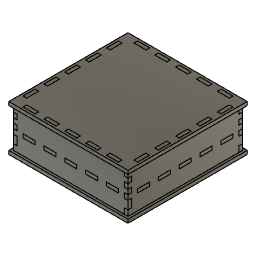
InfinityMirror (Autodesk Fusion 360 design; units mm, degrees)
Autodesk Fusion 360 part; units mm, degrees
sketch "Skizze1" plane through (0, 0, 0) normal (0, 0, 1) x (1, 0, 0) in component "Deckel"
  line L0 (50, -50) -> (-50, -50)
  line L1 (-50, -50) -> (-50, 50)
  line L2 (-50, 50) -> (50, 50)
  line L3 (50, 50) -> (50, -50)
  line L4 (50, -50) -> (-50, 50) construction
  line L5 (-50, -50) -> (50, 50) construction
  line L6 (45, -45) -> (-45, -45) construction
  line L7 (-45, -45) -> (-45, 45) construction
  line L8 (-45, 45) -> (45, 45) construction
  line L9 (45, 45) -> (45, -45) construction
  line L10 (45, -45) -> (-45, 45) construction
  line L11 (-45, -45) -> (45, 45) construction
  line L12 (-40, 45) -> (-30, 45)
  line L13 (-30, 45) -> (-30, 48)
  line L14 (-30, 48) -> (-40, 48)
  line L15 (-40, 48) -> (-40, 45)
  line L16 (-22.5, 45) -> (-12.5, 45)
  line L17 (-12.5, 45) -> (-12.5, 48)
  line L18 (-22.5, 48) -> (-22.5, 45)
  line L19 (-12.5, 48) -> (-22.5, 48)
  line L20 (-5, 45) -> (5, 45)
  line L21 (5, 45) -> (5, 48)
  line L22 (-5, 48) -> (-5, 45)
  line L23 (5, 48) -> (-5, 48)
  line L24 (12.5, 45) -> (22.5, 45)
  line L25 (22.5, 45) -> (22.5, 48)
  line L26 (12.5, 48) -> (12.5, 45)
  line L27 (22.5, 48) -> (12.5, 48)
  line L28 (30, 45) -> (40, 45)
  line L29 (40, 45) -> (40, 48)
  line L30 (30, 48) -> (30, 45)
  line L31 (40, 48) -> (30, 48)
  line L32 (-45, -22.5) -> (-45, -12.5)
  line L33 (-45, -12.5) -> (-48, -12.5)
  line L34 (-48, -12.5) -> (-48, -22.5)
  line L35 (-48, -22.5) -> (-45, -22.5)
  line L36 (-45, -40) -> (-45, -30)
  line L37 (-45, -30) -> (-48, -30)
  line L38 (-48, -40) -> (-45, -40)
  line L39 (-48, -30) -> (-48, -40)
  line L40 (-45, -5) -> (-45, 5)
  line L41 (-45, 5) -> (-48, 5)
  line L42 (-48, -5) -> (-45, -5)
  line L43 (-48, 5) -> (-48, -5)
  line L44 (-45, 12.5) -> (-45, 22.5)
  line L45 (-45, 22.5) -> (-48, 22.5)
  line L46 (-48, 12.5) -> (-45, 12.5)
  line L47 (-48, 22.5) -> (-48, 12.5)
  line L48 (-45, 30) -> (-45, 40)
  line L49 (-45, 40) -> (-48, 40)
  line L50 (-48, 30) -> (-45, 30)
  line L51 (-48, 40) -> (-48, 30)
  line L52 (22.5, -45) -> (12.5, -45)
  line L53 (12.5, -45) -> (12.5, -48)
  line L54 (12.5, -48) -> (22.5, -48)
  line L55 (22.5, -48) -> (22.5, -45)
  line L56 (40, -45) -> (30, -45)
  line L57 (30, -45) -> (30, -48)
  line L58 (40, -48) -> (40, -45)
  line L59 (30, -48) -> (40, -48)
  line L60 (5, -45) -> (-5, -45)
  line L61 (-5, -45) -> (-5, -48)
  line L62 (5, -48) -> (5, -45)
  line L63 (-5, -48) -> (5, -48)
  line L64 (-12.5, -45) -> (-22.5, -45)
  line L65 (-22.5, -45) -> (-22.5, -48)
  line L66 (-12.5, -48) -> (-12.5, -45)
  line L67 (-22.5, -48) -> (-12.5, -48)
  line L68 (-30, -45) -> (-40, -45)
  line L69 (-40, -45) -> (-40, -48)
  line L70 (-30, -48) -> (-30, -45)
  line L71 (-40, -48) -> (-30, -48)
  line L72 (45, 22.5) -> (45, 12.5)
  line L73 (45, 12.5) -> (48, 12.5)
  line L74 (48, 12.5) -> (48, 22.5)
  line L75 (48, 22.5) -> (45, 22.5)
  line L76 (45, 40) -> (45, 30)
  line L77 (45, 30) -> (48, 30)
  line L78 (48, 40) -> (45, 40)
  line L79 (48, 30) -> (48, 40)
  line L80 (45, 5) -> (45, -5)
  line L81 (45, -5) -> (48, -5)
  line L82 (48, 5) -> (45, 5)
  line L83 (48, -5) -> (48, 5)
  line L84 (45, -12.5) -> (45, -22.5)
  line L85 (45, -22.5) -> (48, -22.5)
  line L86 (48, -12.5) -> (45, -12.5)
  line L87 (48, -22.5) -> (48, -12.5)
  line L88 (45, -30) -> (45, -40)
  line L89 (45, -40) -> (48, -40)
  line L90 (48, -30) -> (45, -30)
  line L91 (48, -40) -> (48, -30)
  dimension "d1" = 100
  dimension "d2" = 100
  dimension "d3" = 90
  dimension "d7" = 10
  dimension "d8" = 3
  dimension "d9" = 2
  dimension "d12" = 70
  dimension "d13" = 0
  dimension "d14" = 10
  dimension "d16" = 360
  constraint horizontal L0
  constraint perpendicular L0 L1
  constraint parallel L1 L3
  constraint coincident L4 origin
  constraint coincident L5 origin
  constraint horizontal L6
  constraint perpendicular L6 L7
  constraint parallel L7 L9
  constraint coincident L10 origin
  constraint coincident L11 origin
  constraint coincident L4 L6.start
  constraint horizontal L12
  constraint vertical L13
  constraint horizontal L14
  constraint vertical L15
  constraint coincident L8 L12.start
  measures "d1" distance of L0.start L2.end
  measures "d2" distance of L0.start L0.end
  measures "d3" distance of L6.start L6.end
  measures "d7" distance of L12.start L12.end
  measures "d8" distance of L12.end L13.end
  measures "d9" distance of L2 L14
  measures "d14" distance of L1 L15
extrude "Extrusion1" add sketch "Skizze1" against normal blind 3 makes body 1 in component "Deckel"
sketch "Skizze1 (2)" plane through (0, 0, 0) normal (0, 0, 1) x (-1, 0, 0) in component "Seitenwand"
  line L0 (48, 5) -> (48, -5)
  line L1 (48, -5) -> (45, -5)
  line L2 (45, -5) -> (45, 5)
  line L3 (45, 5) -> (48, 5)
  line L4 (48, -30) -> (48, -40)
  line L5 (48, -40) -> (45, -40)
  line L6 (45, -40) -> (45, -30)
  line L7 (45, -30) -> (48, -30)
  line L8 (48, -12.5) -> (48, -22.5)
  line L9 (48, -22.5) -> (45, -22.5)
  line L10 (45, -22.5) -> (45, -12.5)
  line L11 (45, -12.5) -> (48, -12.5)
  line L12 (-22.5, 45) -> (-22.5, 48)
  line L13 (-22.5, 48) -> (-12.5, 48)
  line L14 (-12.5, 48) -> (-12.5, 45)
  line L15 (-12.5, 45) -> (-22.5, 45)
  line L16 (48, 40) -> (48, 30)
  line L17 (48, 30) -> (45, 30)
  line L18 (45, 30) -> (45, 40)
  line L19 (45, 40) -> (48, 40)
  line L20 (45, 22.5) -> (48, 22.5)
  line L21 (48, 22.5) -> (48, 12.5)
  line L22 (48, 12.5) -> (45, 12.5)
  line L23 (45, 12.5) -> (45, 22.5)
  line L24 (-30, -48) -> (-40, -48)
  line L25 (-40, -48) -> (-40, -45)
  line L26 (-40, -45) -> (-30, -45)
  line L27 (-30, -45) -> (-30, -48)
  line L28 (22.5, -48) -> (12.5, -48)
  line L29 (12.5, -48) -> (12.5, -45)
  line L30 (12.5, -45) -> (22.5, -45)
  line L31 (22.5, -45) -> (22.5, -48)
  line L32 (5, -48) -> (-5, -48)
  line L33 (-5, -48) -> (-5, -45)
  line L34 (-5, -45) -> (5, -45)
  line L35 (5, -45) -> (5, -48)
  line L36 (-12.5, -48) -> (-22.5, -48)
  line L37 (-22.5, -48) -> (-22.5, -45)
  line L38 (-22.5, -45) -> (-12.5, -45)
  line L39 (-12.5, -45) -> (-12.5, -48)
  line L40 (40, -45) -> (40, -48)
  line L41 (40, -48) -> (30, -48)
  line L42 (30, -48) -> (30, -45)
  line L43 (30, -45) -> (40, -45)
  line L44 (-40, 48) -> (-30, 48)
  line L45 (-30, 48) -> (-30, 45)
  line L46 (-30, 45) -> (-40, 45)
  line L47 (-40, 45) -> (-40, 48)
  line L48 (-5, 48) -> (5, 48)
  line L49 (5, 48) -> (5, 45)
  line L50 (5, 45) -> (-5, 45)
  line L51 (-5, 45) -> (-5, 48)
  line L52 (12.5, 48) -> (22.5, 48)
  line L53 (22.5, 48) -> (22.5, 45)
  line L54 (22.5, 45) -> (12.5, 45)
  line L55 (12.5, 45) -> (12.5, 48)
  line L56 (30, 48) -> (40, 48)
  line L57 (40, 48) -> (40, 45)
  line L58 (40, 45) -> (30, 45)
  line L59 (30, 45) -> (30, 48)
  line L60 (-45, -22.5) -> (-48, -22.5)
  line L61 (-48, -22.5) -> (-48, -12.5)
  line L62 (-48, -12.5) -> (-45, -12.5)
  line L63 (-45, -12.5) -> (-45, -22.5)
  line L64 (-48, -40) -> (-48, -30)
  line L65 (-48, -30) -> (-45, -30)
  line L66 (-45, -30) -> (-45, -40)
  line L67 (-45, -40) -> (-48, -40)
  line L68 (-48, -5) -> (-48, 5)
  line L69 (-48, 5) -> (-45, 5)
  line L70 (-45, 5) -> (-45, -5)
  line L71 (-45, -5) -> (-48, -5)
  line L72 (-48, 12.5) -> (-48, 22.5)
  line L73 (-48, 22.5) -> (-45, 22.5)
  line L74 (-45, 22.5) -> (-45, 12.5)
  line L75 (-45, 12.5) -> (-48, 12.5)
  line L76 (-48, 30) -> (-48, 40)
  line L77 (-48, 40) -> (-45, 40)
  line L78 (-45, 40) -> (-45, 30)
  line L79 (-45, 30) -> (-48, 30)
  line L80 (-50, -50) -> (50, -50)
  line L81 (50, -50) -> (50, 50)
  line L82 (50, 50) -> (-50, 50)
  line L83 (-50, 50) -> (-50, -50)
  line L84 (48, 48) -> (-45, 48)
  line L85 (-45, 48) -> (-45, 45)
  line L86 (-45, 45) -> (48, 45)
  line L87 (48, 45) -> (48, 48)
  dimension "d19" = 93
  dimension "d20" = 3
  dimension "d21" = 2
  dimension "d22" = 2
  constraint horizontal L84
  constraint vertical L85
  constraint horizontal L86
  constraint vertical L87
  measures "d19" distance of L84.start L84.end
  measures "d20" distance of L84.end L85.end
  measures "d21" distance of L82 L84
  measures "d22" distance of L81 L87
extrude "Extrusion1'" add sketch "Skizze1 (2)" along normal blind 32.5 separate body contours L12 L45 L84 L86 | L12 L13 L14 L15 L84 L86 | L14 L51 L84 L86 | L44 L45 L46 L47 L84 L86 | L48 L49 L50 L51 L84 L86 | L47 L84 L85 L86 | L49 L55 L84 L86 | L52 L53 L54 L55 L84 L86 | L53 L59 L84 L86 | L56 L57 L58 L59 L84 L86 | L57 L84 L86 L87 makes body 2 in component "Seitenwand"
sketch "Skizze2" plane through (0, 0, 0) normal (0, 0, -1) x (1, 0, 0) in component "Seitenwand"
  line L0 (-48, 48) -> (-48, 45)
  line L1 (-48, 45) -> (45, 45)
  line L2 (45, 45) -> (45, 48)
  line L3 (45, 48) -> (-48, 48)
  line L4 (40, 45) -> (30, 45)
  line L5 (30, 45) -> (30, 48)
  line L6 (30, 48) -> (40, 48)
  line L7 (40, 48) -> (40, 45)
  line L8 (22.5, 48) -> (22.5, 45)
  line L9 (22.5, 45) -> (12.5, 45)
  line L10 (12.5, 48) -> (22.5, 48)
  line L11 (12.5, 45) -> (12.5, 48)
  line L12 (5, 48) -> (5, 45)
  line L13 (5, 45) -> (-5, 45)
  line L14 (-5, 48) -> (5, 48)
  line L15 (-5, 45) -> (-5, 48)
  line L16 (-12.5, 48) -> (-12.5, 45)
  line L17 (-12.5, 45) -> (-22.5, 45)
  line L18 (-22.5, 48) -> (-12.5, 48)
  line L19 (-22.5, 45) -> (-22.5, 48)
  line L20 (-30, 48) -> (-30, 45)
  line L21 (-30, 45) -> (-40, 45)
  line L22 (-40, 48) -> (-30, 48)
  line L23 (-40, 45) -> (-40, 48)
  dimension "d25" = 10
  dimension "d26" = 5
  dimension "d29" = 70
  dimension "d30" = 0
  constraint horizontal L4
  constraint vertical L5
  constraint horizontal L6
  constraint vertical L7
  constraint coincident L3 L5.end
  constraint coincident L1 L4.start
  measures "d25" distance of L5.end L6.end
  measures "d26" distance of L2 L7
extrude "Extrusion2" add sketch "Skizze2" along normal blind 3 contours L1 L3 L20 L21 L22 L23 | L1 L3 L16 L17 L18 L19 | L1 L3 L12 L13 L14 L15 | L1 L3 L8 L9 L10 L11 | L1 L3 L4 L5 L6 L7 bodies 2 in component "Seitenwand"
sketch "Skizze3" plane through (0, 0, 32.5) normal (0, 0, 1) x (-1, 0, 0) in component "Seitenwand"
  line L0 (48, 45) -> (48, 48)
  line L1 (48, 48) -> (-45, 48)
  line L2 (-45, 48) -> (-45, 45)
  line L3 (-45, 45) -> (48, 45)
  line L4 (-40, 48) -> (-30, 48)
  line L5 (-30, 48) -> (-30, 45)
  line L6 (-30, 45) -> (-40, 45)
  line L7 (-40, 45) -> (-40, 48)
  line L8 (-22.5, 48) -> (-12.5, 48)
  line L9 (-12.5, 48) -> (-12.5, 45)
  line L10 (-12.5, 45) -> (-22.5, 45)
  line L11 (-22.5, 45) -> (-22.5, 48)
  line L12 (-5, 48) -> (5, 48)
  line L13 (5, 48) -> (5, 45)
  line L14 (5, 45) -> (-5, 45)
  line L15 (-5, 45) -> (-5, 48)
  line L16 (12.5, 48) -> (22.5, 48)
  line L17 (22.5, 48) -> (22.5, 45)
  line L18 (22.5, 45) -> (12.5, 45)
  line L19 (12.5, 45) -> (12.5, 48)
  line L20 (30, 48) -> (40, 48)
  line L21 (40, 48) -> (40, 45)
  line L22 (40, 45) -> (30, 45)
  line L23 (30, 45) -> (30, 48)
  dimension "d33" = 10
  dimension "d34" = 5
  dimension "d37" = 70
  dimension "d38" = 0
  constraint horizontal L4
  constraint vertical L5
  constraint horizontal L6
  constraint vertical L7
  constraint coincident L3 L5.end
  constraint coincident L1 L4.start
  measures "d33" distance of L5.end L6.end
  measures "d34" distance of L2 L7
extrude "Extrusion3" add sketch "Skizze3" along normal blind 3 contours L1 L3 L20 L21 L22 L23 | L1 L3 L16 L17 L18 L19 | L1 L3 L12 L13 L14 L15 | L1 L3 L8 L9 L10 L11 | L1 L3 L4 L5 L6 L7 bodies 2 in component "Seitenwand"
sketch "Skizze4" plane through (45, 0, 0) normal (1, 0, 0) x (0, 1, 0) in component "Seitenwand"
  line L0 (-48, 0) -> (-45, 0)
  line L1 (-45, 0) -> (-45, 32.5)
  line L2 (-45, 32.5) -> (-48, 32.5)
  line L3 (-48, 32.5) -> (-48, 0)
  line L4 (-48, 27.75) -> (-45, 27.75)
  line L5 (-45, 27.75) -> (-45, 23.75)
  line L6 (-45, 23.75) -> (-48, 23.75)
  line L7 (-48, 23.75) -> (-48, 27.75)
  line L8 (-45, 19.75) -> (-45, 15.75)
  line L9 (-45, 15.75) -> (-48, 15.75)
  line L10 (-48, 15.75) -> (-48, 19.75)
  line L11 (-48, 19.75) -> (-45, 19.75)
  line L12 (-48, 11.75) -> (-45, 11.75)
  line L13 (-45, 11.75) -> (-45, 4.75)
  line L14 (-45, 4.75) -> (-48, 4.75)
  line L15 (-48, 4.75) -> (-48, 11.75)
  dimension "d41" = 4
  dimension "d42" = 4.75
  dimension "d45" = 8
  dimension "d46" = 0
  dimension "d93" = 4
  dimension "d94" = 7
  constraint horizontal L4
  constraint vertical L5
  constraint horizontal L6
  constraint vertical L7
  constraint coincident L1 L5.end
  constraint coincident L3 L4.start
  constraint horizontal L12
  constraint vertical L13
  constraint horizontal L14
  constraint vertical L15
  constraint coincident L1 L13.end
  constraint coincident L3 L12.start
  measures "d41" distance of L4.start L6.end
  measures "d42" distance of L2 L4
  measures "d93" distance of L9 L12
  measures "d94" distance of L12.end L13.end
extrude "Extrusion4" add sketch "Skizze4" along normal blind 3 contours L1 L3 L12 L13 L14 L15 | L1 L3 L8 L9 L10 L11 | L1 L3 L4 L5 L6 L7 bodies 2 in component "Seitenwand"
sketch "Skizze5" plane through (-48, 0, 0) normal (-1, 0, 0) x (0, -1, 0) in component "Seitenwand"
  line L0 (45, 0) -> (48, 0)
  line L1 (48, 0) -> (48, 32.5)
  line L2 (48, 32.5) -> (45, 32.5)
  line L3 (45, 32.5) -> (45, 0)
  line L4 (45, 27.75) -> (48, 27.75)
  line L5 (48, 27.75) -> (48, 23.75)
  line L6 (48, 23.75) -> (45, 23.75)
  line L7 (45, 23.75) -> (45, 27.75)
  line L8 (48, 15.75) -> (45, 15.75)
  line L9 (45, 15.75) -> (45, 19.75)
  line L10 (45, 19.75) -> (48, 19.75)
  line L11 (48, 19.75) -> (48, 15.75)
  line L12 (45, 11.75) -> (48, 11.75)
  line L13 (48, 11.75) -> (48, 4.75)
  line L14 (48, 4.75) -> (45, 4.75)
  line L15 (45, 4.75) -> (45, 11.75)
  dimension "d49" = 4
  dimension "d50" = 4.75
  dimension "d53" = 8
  dimension "d54" = 0
  dimension "d95" = 4
  dimension "d96" = 7
  constraint horizontal L4
  constraint vertical L5
  constraint horizontal L6
  constraint vertical L7
  constraint coincident L1 L5.end
  constraint coincident L3 L4.start
  constraint horizontal L12
  constraint vertical L13
  constraint horizontal L14
  constraint vertical L15
  constraint coincident L1 L13.end
  constraint coincident L3 L12.start
  measures "d49" distance of L4.end L5.end
  measures "d50" distance of L2 L4
  measures "d95" distance of L8 L12
  measures "d96" distance of L12.end L13.end
extrude "Extrusion5" cut sketch "Skizze5" against normal blind 3 contours L1 L3 L12 L13 L14 L15 | L1 L3 L8 L9 L10 L11 | L1 L3 L4 L5 L6 L7 bodies 2 in component "Seitenwand"
sketch "Skizze6" plane through (0, -48, 0) normal (0, -1, 0) x (1, 0, 0) in component "Seitenwand"
  line L0 (-45, 23.75) -> (-48, 23.75)
  line L1 (-48, 23.75) -> (-48, 19.75)
  line L2 (-48, 19.75) -> (-45, 19.75)
  line L3 (-45, 19.75) -> (-45, 15.75)
  line L4 (-45, 15.75) -> (-48, 15.75)
  line L5 (-48, 4.75) -> (-48, 0)
  line L6 (-48, 0) -> (-40, 0)
  line L7 (-40, 0) -> (-40, -3)
  line L8 (-40, -3) -> (-30, -3)
  line L9 (-30, -3) -> (-30, 0)
  line L10 (-30, 0) -> (-22.5, 0)
  line L11 (-22.5, 0) -> (-22.5, -3)
  line L12 (-22.5, -3) -> (-12.5, -3)
  line L13 (-12.5, -3) -> (-12.5, 0)
  line L14 (-12.5, 0) -> (-5, 0)
  line L15 (-5, 0) -> (-5, -3)
  line L16 (-5, -3) -> (5, -3)
  line L17 (5, -3) -> (5, 0)
  line L18 (5, 0) -> (12.5, 0)
  line L19 (12.5, 0) -> (12.5, -3)
  line L20 (12.5, -3) -> (22.5, -3)
  line L21 (22.5, -3) -> (22.5, 0)
  line L22 (22.5, 0) -> (30, 0)
  line L23 (30, 0) -> (30, -3)
  line L24 (30, -3) -> (40, -3)
  line L25 (40, -3) -> (40, 0)
  line L26 (40, 0) -> (45, 0)
  line L27 (45, 0) -> (45, 4.75)
  line L28 (48, 4.75) -> (48, 11.75)
  line L29 (45, 15.75) -> (48, 15.75)
  line L30 (48, 15.75) -> (48, 19.75)
  line L31 (48, 19.75) -> (45, 19.75)
  line L32 (45, 19.75) -> (45, 23.75)
  line L33 (45, 23.75) -> (48, 23.75)
  line L34 (48, 23.75) -> (48, 27.75)
  line L35 (48, 27.75) -> (45, 27.75)
  line L36 (45, 27.75) -> (45, 32.5)
  line L37 (45, 32.5) -> (40, 32.5)
  line L38 (40, 32.5) -> (40, 35.5)
  line L39 (40, 35.5) -> (30, 35.5)
  line L40 (30, 35.5) -> (30, 32.5)
  line L41 (30, 32.5) -> (22.5, 32.5)
  line L42 (22.5, 32.5) -> (22.5, 35.5)
  line L43 (22.5, 35.5) -> (12.5, 35.5)
  line L44 (12.5, 35.5) -> (12.5, 32.5)
  line L45 (12.5, 32.5) -> (5, 32.5)
  line L46 (5, 32.5) -> (5, 35.5)
  line L47 (5, 35.5) -> (-5, 35.5)
  line L48 (-5, 35.5) -> (-5, 32.5)
  line L49 (-5, 32.5) -> (-12.5, 32.5)
  line L50 (-12.5, 32.5) -> (-12.5, 35.5)
  line L51 (-12.5, 35.5) -> (-22.5, 35.5)
  line L52 (-22.5, 35.5) -> (-22.5, 32.5)
  line L53 (-22.5, 32.5) -> (-30, 32.5)
  line L54 (-30, 32.5) -> (-30, 35.5)
  line L55 (-30, 35.5) -> (-40, 35.5)
  line L56 (-40, 35.5) -> (-40, 32.5)
  line L57 (-40, 32.5) -> (-48, 32.5)
  line L58 (-48, 32.5) -> (-48, 27.75)
  line L59 (-48, 27.75) -> (-45, 27.75)
  line L60 (-45, 27.75) -> (-45, 23.75)
  line L61 (-40, 16) -> (-30, 16)
  line L62 (-30, 16) -> (-30, 13)
  line L63 (-30, 13) -> (-40, 13)
  line L64 (-40, 13) -> (-40, 16)
  line L65 (-12.5, 13) -> (-22.5, 13)
  line L66 (-22.5, 13) -> (-22.5, 16)
  line L67 (-22.5, 16) -> (-12.5, 16)
  line L68 (-12.5, 16) -> (-12.5, 13)
  line L69 (5, 13) -> (-5, 13)
  line L70 (-5, 13) -> (-5, 16)
  line L71 (-5, 16) -> (5, 16)
  line L72 (5, 16) -> (5, 13)
  line L73 (22.5, 13) -> (12.5, 13)
  line L74 (12.5, 13) -> (12.5, 16)
  line L75 (12.5, 16) -> (22.5, 16)
  line L76 (22.5, 16) -> (22.5, 13)
  line L77 (40, 13) -> (30, 13)
  line L78 (30, 13) -> (30, 16)
  line L79 (30, 16) -> (40, 16)
  line L80 (40, 16) -> (40, 13)
  line L81 (45, 4.75) -> (48, 4.75)
  line L82 (48, 11.75) -> (45, 11.75)
  line L83 (45, 11.75) -> (45, 15.75)
  line L84 (-48, 15.75) -> (-48, 11.75)
  line L85 (-48, 11.75) -> (-45, 11.75)
  line L86 (-45, 11.75) -> (-45, 4.75)
  line L87 (-45, 4.75) -> (-48, 4.75)
  dimension "d59" = 13
  dimension "d60" = 3
  dimension "d61" = 10
  dimension "d62" = 5
  dimension "d65" = 70
  dimension "d66" = 0
  constraint horizontal L61
  constraint vertical L62
  constraint horizontal L63
  constraint vertical L64
  measures "d59" distance of L10 L63
  measures "d60" distance of L61.end L62.end
  measures "d61" distance of L62.end L63.end
  measures "d62" distance of L3 L64
extrude "Extrusion6" cut sketch "Skizze6" against normal blind 3 contours L61 L62 L63 L64 | L65 L66 L67 L68 | L69 L70 L71 L72 | L73 L74 L75 L76 | L77 L78 L79 L80 bodies 2 in component "Seitenwand"
pattern_circular "C-Anordnung1" count 4 over 360 about axis through (0, 0, 1.75) along (0, 0, 1) of bodies 2 makes body 3 at (48, -33.3333, 27) makes body 4 at (33.3333, 48, 27) makes body 5 at (-48, 33.3333, 27) in component "Seitenwand"
sketch "Skizze1 (3)" plane through (0, 0, 0) normal (0, 0, 1) x (-1, 0, 0) in component "Zwischenboden"
  line L0 (48, 5) -> (48, -5)
  line L1 (48, -5) -> (45, -5)
  line L2 (45, -5) -> (45, 5) construction
  line L3 (45, 5) -> (48, 5)
  line L4 (48, -30) -> (48, -40)
  line L5 (48, -40) -> (45, -40)
  line L6 (45, -40) -> (45, -30) construction
  line L7 (45, -30) -> (48, -30)
  line L8 (48, -12.5) -> (48, -22.5)
  line L9 (48, -22.5) -> (45, -22.5)
  line L10 (45, -22.5) -> (45, -12.5) construction
  line L11 (45, -12.5) -> (48, -12.5)
  line L12 (-22.5, 45) -> (-22.5, 48)
  line L13 (-22.5, 48) -> (-12.5, 48)
  line L14 (-12.5, 48) -> (-12.5, 45)
  line L15 (-12.5, 45) -> (-22.5, 45) construction
  line L16 (48, 40) -> (48, 30)
  line L17 (48, 30) -> (45, 30)
  line L18 (45, 30) -> (45, 40) construction
  line L19 (45, 40) -> (48, 40)
  line L20 (45, 22.5) -> (48, 22.5)
  line L21 (48, 22.5) -> (48, 12.5)
  line L22 (48, 12.5) -> (45, 12.5)
  line L23 (45, 12.5) -> (45, 22.5) construction
  line L24 (-30, -48) -> (-40, -48)
  line L25 (-40, -48) -> (-40, -45)
  line L26 (-40, -45) -> (-30, -45) construction
  line L27 (-30, -45) -> (-30, -48)
  line L28 (22.5, -48) -> (12.5, -48)
  line L29 (12.5, -48) -> (12.5, -45)
  line L30 (12.5, -45) -> (22.5, -45) construction
  line L31 (22.5, -45) -> (22.5, -48)
  line L32 (5, -48) -> (-5, -48)
  line L33 (-5, -48) -> (-5, -45)
  line L34 (-5, -45) -> (5, -45) construction
  line L35 (5, -45) -> (5, -48)
  line L36 (-12.5, -48) -> (-22.5, -48)
  line L37 (-22.5, -48) -> (-22.5, -45)
  line L38 (-22.5, -45) -> (-12.5, -45) construction
  line L39 (-12.5, -45) -> (-12.5, -48)
  line L40 (40, -45) -> (40, -48)
  line L41 (40, -48) -> (30, -48)
  line L42 (30, -48) -> (30, -45)
  line L43 (30, -45) -> (40, -45) construction
  line L44 (-40, 48) -> (-30, 48)
  line L45 (-30, 48) -> (-30, 45)
  line L46 (-30, 45) -> (-40, 45) construction
  line L47 (-40, 45) -> (-40, 48)
  line L48 (-5, 48) -> (5, 48)
  line L49 (5, 48) -> (5, 45)
  line L50 (5, 45) -> (-5, 45) construction
  line L51 (-5, 45) -> (-5, 48)
  line L52 (12.5, 48) -> (22.5, 48)
  line L53 (22.5, 48) -> (22.5, 45)
  line L54 (22.5, 45) -> (12.5, 45) construction
  line L55 (12.5, 45) -> (12.5, 48)
  line L56 (30, 48) -> (40, 48)
  line L57 (40, 48) -> (40, 45)
  line L58 (40, 45) -> (30, 45) construction
  line L59 (30, 45) -> (30, 48)
  line L60 (-45, -22.5) -> (-48, -22.5)
  line L61 (-48, -22.5) -> (-48, -12.5)
  line L62 (-48, -12.5) -> (-45, -12.5)
  line L63 (-45, -12.5) -> (-45, -22.5) construction
  line L64 (-48, -40) -> (-48, -30)
  line L65 (-48, -30) -> (-45, -30)
  line L66 (-45, -30) -> (-45, -40) construction
  line L67 (-45, -40) -> (-48, -40)
  line L68 (-48, -5) -> (-48, 5)
  line L69 (-48, 5) -> (-45, 5)
  line L70 (-45, 5) -> (-45, -5) construction
  line L71 (-45, -5) -> (-48, -5)
  line L72 (-48, 12.5) -> (-48, 22.5)
  line L73 (-48, 22.5) -> (-45, 22.5)
  line L74 (-45, 22.5) -> (-45, 12.5) construction
  line L75 (-45, 12.5) -> (-48, 12.5)
  line L76 (-48, 30) -> (-48, 40)
  line L77 (-48, 40) -> (-45, 40)
  line L78 (-45, 40) -> (-45, 30) construction
  line L79 (-45, 30) -> (-48, 30)
  line L80 (-50, -50) -> (50, -50)
  line L81 (50, -50) -> (50, 50)
  line L82 (50, 50) -> (-50, 50)
  line L83 (-50, 50) -> (-50, -50)
  line L84 (-45, -45) -> (45, 45) construction
  line L85 (45, -45) -> (-45, 45) construction
  line L86 (30, 45) -> (30, 48)
  line L87 (30, 48) -> (40, 48)
  line L88 (40, 48) -> (40, 45)
  line L89 (45, 45) -> (40, 45)
  line L90 (22.5, 48) -> (22.5, 45)
  line L91 (12.5, 48) -> (22.5, 48)
  line L92 (12.5, 45) -> (12.5, 48)
  line L93 (5, 48) -> (5, 45)
  line L94 (-5, 48) -> (5, 48)
  line L95 (-5, 45) -> (-5, 48)
  line L96 (-12.5, 48) -> (-12.5, 45)
  line L97 (-22.5, 48) -> (-12.5, 48)
  line L98 (-22.5, 45) -> (-22.5, 48)
  line L99 (-30, 48) -> (-30, 45)
  line L100 (-40, 48) -> (-30, 48)
  line L101 (-40, 45) -> (-40, 48)
  line L102 (30, 45) -> (22.5, 45)
  line L103 (12.5, 45) -> (5, 45)
  line L104 (-5, 45) -> (-12.5, 45)
  line L105 (-22.5, 45) -> (-30, 45)
  line L106 (-40, 45) -> (-45, 45)
  line L107 (-45, 30) -> (-48, 30)
  line L108 (-48, 30) -> (-48, 40)
  line L109 (-48, 40) -> (-45, 40)
  line L110 (-45, 12.5) -> (-48, 12.5)
  line L111 (-48, 22.5) -> (-45, 22.5)
  line L112 (-48, 12.5) -> (-48, 22.5)
  line L113 (-45, -5) -> (-48, -5)
  line L114 (-48, 5) -> (-45, 5)
  line L115 (-48, -5) -> (-48, 5)
  line L116 (-45, -22.5) -> (-48, -22.5)
  line L117 (-48, -12.5) -> (-45, -12.5)
  line L118 (-48, -22.5) -> (-48, -12.5)
  line L119 (-45, -40) -> (-48, -40)
  line L120 (-48, -30) -> (-45, -30)
  line L121 (-48, -40) -> (-48, -30)
  line L122 (-30, -45) -> (-30, -48)
  line L123 (-30, -48) -> (-40, -48)
  line L124 (-40, -48) -> (-40, -45)
  line L125 (-12.5, -45) -> (-12.5, -48)
  line L126 (-22.5, -48) -> (-22.5, -45)
  line L127 (-12.5, -48) -> (-22.5, -48)
  line L128 (5, -45) -> (5, -48)
  line L129 (-5, -48) -> (-5, -45)
  line L130 (5, -48) -> (-5, -48)
  line L131 (22.5, -45) -> (22.5, -48)
  line L132 (12.5, -48) -> (12.5, -45)
  line L133 (22.5, -48) -> (12.5, -48)
  line L134 (40, -45) -> (40, -48)
  line L135 (30, -48) -> (30, -45)
  line L136 (40, -48) -> (30, -48)
  line L137 (45, -30) -> (48, -30)
  line L138 (48, -30) -> (48, -40)
  line L139 (48, -40) -> (45, -40)
  line L140 (45, -12.5) -> (48, -12.5)
  line L141 (48, -22.5) -> (45, -22.5)
  line L142 (48, -12.5) -> (48, -22.5)
  line L143 (45, 5) -> (48, 5)
  line L144 (48, -5) -> (45, -5)
  line L145 (48, 5) -> (48, -5)
  line L146 (45, 22.5) -> (48, 22.5)
  line L147 (48, 12.5) -> (45, 12.5)
  line L148 (48, 22.5) -> (48, 12.5)
  line L149 (45, 40) -> (48, 40)
  line L150 (48, 30) -> (45, 30)
  line L151 (48, 40) -> (48, 30)
  line L152 (-45, 45) -> (-45, 40)
  line L153 (-45, 30) -> (-45, 22.5)
  line L154 (-45, 12.5) -> (-45, 5)
  line L155 (-45, -5) -> (-45, -12.5)
  line L156 (-45, -22.5) -> (-45, -30)
  line L157 (-45, -40) -> (-45, -45)
  line L158 (-45, -45) -> (-40, -45)
  line L159 (-30, -45) -> (-22.5, -45)
  line L160 (-12.5, -45) -> (-5, -45)
  line L161 (5, -45) -> (12.5, -45)
  line L162 (22.5, -45) -> (30, -45)
  line L163 (45, -30) -> (45, -22.5)
  line L164 (45, -12.5) -> (45, -5)
  line L165 (45, 5) -> (45, 12.5)
  line L166 (45, 22.5) -> (45, 30)
  line L167 (45, 40) -> (45, 45)
  line L168 (45, -40) -> (40, -45)
  dimension "d69" = 90
  dimension "d70" = 90
  dimension "d71" = 10
  dimension "d74" = 70
  dimension "d75" = 0
  dimension "d77" = 360
  dimension "d92" = 7.0711
  constraint horizontal L158
  constraint parallel L89 L158
  constraint coincident L84 origin
  constraint coincident L85 origin
  constraint vertical L86
  constraint horizontal L87
  constraint vertical L88
  constraint coincident L56.start L59.end
  constraint coincident L58 L57.end
  constraint collinear L89 L102
  constraint collinear L102 L103
  constraint collinear L103 L104
  constraint collinear L104 L105
  constraint collinear L105 L106
  constraint collinear L152 L153
  constraint collinear L153 L154
  constraint collinear L154 L155
  constraint collinear L155 L156
  constraint collinear L156 L157
  constraint collinear L158 L159
  constraint collinear L159 L160
  constraint collinear L160 L161
  constraint collinear L161 L162
  constraint collinear L163 L164
  constraint collinear L164 L165
  constraint collinear L165 L166
  constraint collinear L166 L167
  constraint coincident L5.end L6.start
  measures "d69" distance of L84.end L85.end
  measures "d70" distance of L85.start L84.end
  measures "d71" distance of L56.start L56.end
  measures "d92" distance of L40.start L5.end
extrude "Extrusion1''" add sketch "Skizze1 (3)" along normal blind 3 from surface at 13 separate body contours L0 L1 L3 L4 L5 L7 L8 L9 L11 L12 L13 L14 L16 L17 L19 L20 L21 L22 L24 L25 L27 L28 L29 L31 L32 L33 L35 L36 L37 L39 L40 L41 L42 L44 L45 L47 L48 L49 L51 L52 L53 L55 L56 L57 L59 L60 L61 L62 L64 L65 L67 L68 L69 L71 L72 L73 L75 L76 L77 L79 L86 L87 L88 L89 L90 L91 L92 L93 L94 L95 L96 L97 L98 L99 L100 L101 L102 L103 L104 L105 L106 L107 L108 L109 L110 L111 L112 L113 L114 L115 L116 L117 L118 L119 L120 L121 L122 L123 L124 L125 L126 L127 L128 L129 L130 L131 L132 L133 L134 L135 L136 L137 L138 L139 L140 L141 L142 L143 L144 L145 L146 L147 L148 L149 L150 L151 L152 L153 L154 L155 L156 L157 L158 L159 L160 L161 L162 L163 L164 L165 L166 L167 L168 makes body 6 in component "Zwischenboden"
pattern_linear "00000000-0000-0000-0000-000000000000" [suppressed]
extrude "Extrusion2'" [suppressed] in component "Zwischenboden"
component "Deckel" placed x (1, 0, 0) y (0, 1, 0) z (0, 0, 1) at (0, 0, 0)
component "Seitenwand" placed x (1, 0, 0) y (0, 1, 0) z (0, 0, 1) at (0, 0, 0)
component "Zwischenboden" placed x (1, 0, 0) y (0, 1, 0) z (0, 0, 1) at (0, 0, 0)
component "Deckel" placed x (1, 0, 0) y (0, 1, 0) z (0, 0, 1) at (0, 0, 35.5)
